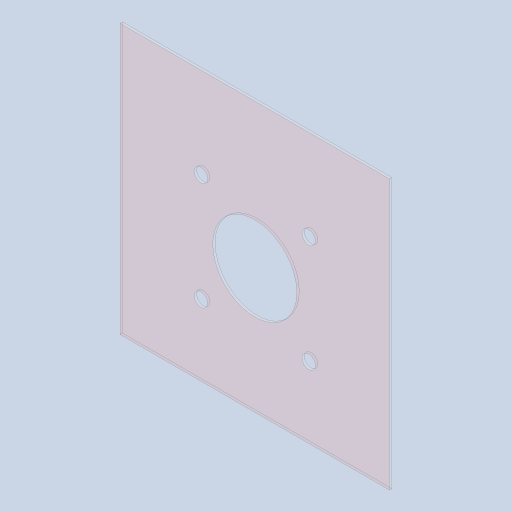
# Autodesk Inventor part: cage_wall_back
Saved by Autodesk Inventor 2024.4 (Build 284460030, 460C)
## iProperties
Created: 2026-03-25
Part Number: cage_wall_back
Material: Generic
Document SubType Name: Modeling
Designer: tooles01
Density: 1 g/cm^3
Appearance: Clear - Light
Author: tooles01
Autodesk Inventor part; units mm, degrees
ref_plane "YZ Plane" through (0, 0, 0) normal (1, 0, 0) x (0, 1, 0)
ref_plane "XZ Plane" through (0, 0, 0) normal (0, 1, 0) x (-1, 0, 0)
ref_plane "XY Plane" through (0, 0, 0) normal (0, 0, 1) x (1, 0, 0)
sketch "Sketch1" plane through (0, 0, 0) normal (0, 0, 1) x (1, 0, 0)
  line L0 (-3.4369, 182.883) -> (196.5631, 182.883)
  line L1 (196.5631, 182.883) -> (196.5631, 42.883)
  line L2 (196.5631, 42.883) -> (-3.4369, 42.883)
  line L3 (-3.4369, 42.883) -> (-3.4369, 182.883)
  circle A0 centre (96.5631, 79.883) radius 12.5
  line L4 (-3.4369, 122.883) -> (196.5631, 122.883)
  line L5 (136.5631, 122.883) -> (136.5631, 42.883)
  line L6 (56.5631, 122.883) -> (56.5631, 42.883)
  circle A1 centre (80.5631, 95.883) radius 2
  circle A2 centre (112.5631, 95.883) radius 2
  circle A3 centre (80.5631, 63.883) radius 2
  circle A4 centre (112.5631, 63.883) radius 2
  line L7 (80.5631, 95.883) -> (112.5631, 95.883) construction
  line L8 (112.5631, 95.883) -> (112.5631, 63.883) construction
  line L9 (112.5631, 63.883) -> (80.5631, 63.883) construction
  line L10 (80.5631, 63.883) -> (80.5631, 95.883) construction
  point P0 (0, 0)
  point P1 (96.5631, 42.883)
  point P2 (96.5631, 95.883)
  point P3 (80.5631, 79.883)
  dimension "d0" = 140
  dimension "d1" = 200
  dimension "d2" = 25
  dimension "d5" = 80
  dimension "d6" = 60
  dimension "d7" = 60
  dimension "d8" = 37
  dimension "d9" = 4
  dimension "d10" = 32
  dimension "d11" = 32
  dimension "d12" = 40
  dimension "d13" = 80
  constraints: 22 end point, 6 perpendicular, 6 point on line, 5 centre point, 4 coincident, 3 equal radius, 3 midpoint, 2 horizontal, 2 vertical alignment, 1 horizontal alignment, 1 other
  measures "d0" distance of L2.end L0.start
  measures "d1" distance of L0.start L0.end
  measures "d2" diameter of A0
  measures "d5" distance between parallel lines of L2 L4
  measures "d6" distance between parallel lines of L3 L6
  measures "d7" distance between parallel lines of L1 L5
  measures "d8" distance from line of L2 A0.centre
  measures "d9" diameter of A1
  measures "d10" distance of L8.end L9.end
  measures "d11" distance of L9.end L7.start
  measures "d12" distance from line of L6 A0.centre
  measures "d13" distance between parallel lines of L5 L6
extrude "Extrusion1" add sketch "Sketch1" against normal blind 0.7 contours L4 L5 L2 L6
equation "\"d7\" = d6"
body "Solid1"
